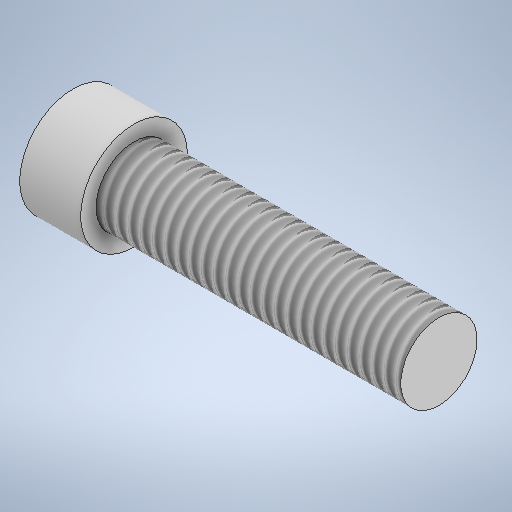
# Autodesk Inventor part: fastener
Saved by Autodesk Inventor 2025.1 (Build 291241000, 241)
## iProperties
Created: 2024-09-02
Part Number: fastener
Material: Generisch
Document SubType Name: Modeling
Designer: ffogue
Density: 1 g/cm^3
Appearance: Vorgabe
Author: ffogue
Autodesk Inventor part; units mm, degrees
ref_plane "YZ Plane" through (0, 0, 0) normal (1, 0, 0) x (0, 1, 0)
ref_plane "XZ Plane" through (0, 0, 0) normal (0, 1, 0) x (-1, 0, 0)
ref_plane "XY Plane" through (0, 0, 0) normal (0, 0, 1) x (1, 0, 0)
sketch "Sketch1" plane through (0, 0, 0) normal (0, 0, 1) x (1, 0, 0)
  line L0 (0, 0) -> (0, 3.5)
  line L1 (0, 3.5) -> (4, 3.5)
  line L2 (4, 3.5) -> (4, 2.5)
  line L3 (4, 2.5) -> (24, 2.5)
  line L4 (24, 2.5) -> (24, 0)
  line L5 (24, 0) -> (0, 0)
  dimension "d0" = 24
  dimension "d1" = 20
  dimension "d2" = 5
  dimension "d3" = 7
  constraints: 12 end point, 5 perpendicular, 1 vertical
  measures "d0" distance of L4.end L0.start
  measures "d1" distance of L2.end L3.end
  measures "d2" diameter of L3 L5
  measures "d3" diameter of L1 L5
revolve "Revolution1" add sketch "Sketch1" angle 360 about axis through (24, 0, 0) along (-1, 0, 0)
thread "Thread1" size "M5x0.8" class "6g" standard "ISO Metric profile" full length
body "Solid1"
